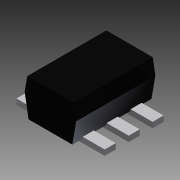
# Autodesk Inventor part: DualSchmittTrig
Saved by Autodesk Inventor 2014 (Build 180170000, 170)
## iProperties
Created: 2015-11-06
Part Number: DualSchmittTrig
Material: Generic
Document SubType Name: Modeling
Designer: Owner
Density: 1 g/cm^3
Appearance: Default
Author: Owner
Autodesk Inventor part; units mm, degrees
ref_plane "YZ Plane" through (0, 0, 0) normal (1, 0, 0) x (0, 1, 0)
ref_plane "XZ Plane" through (0, 0, 0) normal (0, 1, 0) x (-1, 0, 0)
sketch "Sketch1" plane through (0, 0, 0) normal (0, 0, 1) x (1, 0, 0)
  line L0 (-0.7979, 0.6612) -> (0.6021, 0.6612)
  line L1 (0.6021, 0.6612) -> (0.6021, -0.3388)
  line L2 (0.6021, -0.3388) -> (-0.7979, -0.3388)
  line L3 (-0.7979, -0.3388) -> (-0.7979, 0.6612)
  line L4 (-0.7979, 0.2612) -> (0.6021, 0.2612)
  line L5 (-0.7274, 0.6612) -> (-0.7979, 0.2612)
  line L6 (-0.7979, 0.2612) -> (-0.6921, -0.3388)
  line L7 (0.6021, 0.2612) -> (0.4963, -0.3388)
  line L8 (0.6021, 0.2612) -> (0.5316, 0.6612)
  point P0 (0, 0)
  dimension "d0" = 1.4
  dimension "d1" = 1
  dimension "d2" = 0.4
  dimension "d3" = 10
  dimension "d4" = 10
  dimension "d5" = 10
  constraints: 18 end point, 6 point on line, 3 parallel, 2 perpendicular, 1 horizontal
  measures "d0" distance of L0.start L0.end
  measures "d1" distance of L0.end L1.end
  measures "d2" distance between parallel lines of L0 L4
  measures "d3" angle of L3 L5
  measures "d4" angle of L1 L8
  measures "d5" angle of L3 L6
extrude "Extrusion1" add sketch "Sketch1" along normal blind 2.15 contours L0 L8 L4 L5 | L4 L7 L2 L6
ref_plane "Work Plane1" through (0, 0, 1.725) normal (0, 0, 1) x (1, 0, 0)
sketch "Sketch2" plane through (0, 0, 1.725) normal (0, 0, 1) x (1, 0, 0)
  line L0 (-1.2978, -0.2888) -> (1.1022, -0.2888)
  line L1 (1.1022, -0.2888) -> (1.1022, -0.4388)
  line L2 (1.1022, -0.4388) -> (-1.2978, -0.4388)
  line L3 (-1.2978, -0.4388) -> (-1.2978, -0.2888)
  line L4 (0.5316, 0.6612) -> (-0.7274, 0.6612) projected
  point P0 (0, 0)
  dimension "d9" = 1.1
  dimension "d10" = 0.15
  dimension "d11" = 2.4
  constraints: 8 end point, 2 parallel, 1 horizontal, 1 perpendicular
  measures "d9" distance between parallel lines of L2 L4
  measures "d10" distance of L0.end L1.end
  measures "d11" distance of L1.end L2.end
extrude "Extrusion2" add sketch "Sketch2" along normal mid plane 0.3
pattern_linear "Rectangular Pattern1" count 3 spacing 0.65 along (0, 0, -1) of "Extrusion2"
body "Solid1"
